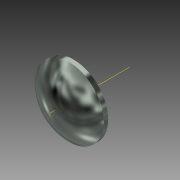
# Autodesk Inventor part: Melles Griot 01MCG023 Spherical Mirror
Saved by Autodesk Inventor 2015 (Build 190159000, 159)
## iProperties
Created: 2014-07-17
Part Number: Melles Griot 01MCG023 Spherical Mirror
Material: Mirror
Document SubType Name: Modeling
Designer: I Rabey
Density: 2.18 g/cm^3
Appearance: Basic
Author: I Rabey
Autodesk Inventor part; units mm, degrees
ref_plane "YZ Plane" through (0, 0, 0) normal (1, 0, 0) x (0, 1, 0)
ref_plane "XZ Plane" through (0, 0, 0) normal (0, 1, 0) x (-1, 0, 0)
ref_plane "XY Plane" through (0, 0, 0) normal (0, 0, 1) x (1, 0, 0)
sketch "Sketch3" plane through (0, 0, 0) normal (0, 0, 1) x (1, 0, 0)
  arc A0 (60, 0) -> (-60, 0) centre (0, 0) ccw
  line L0 (0, 0) -> (60, 0) construction
  line L1 (0, 0) -> (-60, 0) construction
  arc A1 (64, 0) -> (-64, 0) centre (0, 0) ccw
  line L2 (0, 0) -> (64, 0) construction
  line L3 (0, 0) -> (-64, 0) construction
  line L4 (-60, 0) -> (-64, 0)
  line L5 (64, 0) -> (60, 0)
  line L6 (-89.6, 0) -> (89.6, 0) projected
  dimension "d4" = 60
  dimension "d5" = 180
  dimension "d6" = 64
  dimension "d7" = 180
  constraints: 12 end point, 4 point on circle, 2 centre point, 2 coincident, 1 collinear
  measures "d4" radius of A0
  measures "d5" angle of L1 L0
  measures "d6" radius of A1
  measures "d7" angle of L3 L2
revolve "Revolution1" add sketch "Sketch3" angle 180 about axis through (-10, 0, 0) along (1, 0, 0) contours A0 L4 A1 L5
sketch "Sketch4" plane through (0, 0, 0) normal (0, 0, 1) x (1, 0, 0)
  circle A0 centre (0, 0) radius 64
  circle A1 centre (0, 0) radius 45
  dimension "d9" = 128
  dimension "d10" = 90
  constraints: 2 centre point, 2 coincident
  measures "d9" diameter of A0
  measures "d10" diameter of A1
extrude "Extrusion1" cut sketch "Sketch4" along normal blind 50
body "Solid1"
